Autodesk Fusion 360 part; units mm, degrees
(part 2 of 2)
sketch "Sketch9" plane through (0, 0, 3) normal (0, 0, 1) x (-1, 0, 0)
  line L0 (-28.8135, -26) -> (-30.5455, -23)
  line L1 (-30.5455, -23) -> (-28.8135, -20)
  line L2 (-28.8135, -20) -> (-25.3494, -20)
  line L3 (-25.3494, -20) -> (-23.6173, -23)
  line L4 (-23.6173, -23) -> (-25.3494, -26)
  line L5 (-25.3494, -26) -> (-28.8135, -26)
  line L6 (-28.8135, -33) -> (-30.5455, -30)
  line L7 (-30.5455, -30) -> (-28.8135, -27)
  line L8 (-28.8135, -27) -> (-25.3494, -27)
  line L9 (-25.3494, -27) -> (-23.6173, -30)
  line L10 (-23.6173, -30) -> (-25.3494, -33)
  line L11 (-25.3494, -33) -> (-28.8135, -33)
  line L12 (-34.8756, -29.5) -> (-36.6077, -26.5)
  line L13 (-36.6077, -26.5) -> (-34.8756, -23.5)
  line L14 (-34.8756, -23.5) -> (-31.4115, -23.5)
  line L15 (-31.4115, -23.5) -> (-29.6795, -26.5)
  line L16 (-29.6795, -26.5) -> (-31.4115, -29.5)
  line L17 (-31.4115, -29.5) -> (-34.8756, -29.5)
  line L18 (-40.9378, -26) -> (-42.6699, -23)
  line L19 (-42.6699, -23) -> (-40.9378, -20)
  line L20 (-40.9378, -20) -> (-37.4737, -20)
  line L21 (-37.4737, -20) -> (-35.7417, -23)
  line L22 (-35.7417, -23) -> (-37.4737, -26)
  line L23 (-37.4737, -26) -> (-40.9378, -26)
  line L24 (-34.8756, -22.5) -> (-36.6077, -19.5)
  line L25 (-36.6077, -19.5) -> (-34.8756, -16.5)
  line L26 (-34.8756, -16.5) -> (-31.4115, -16.5)
  line L27 (-31.4115, -16.5) -> (-29.6795, -19.5)
  line L28 (-29.6795, -19.5) -> (-31.4115, -22.5)
  line L29 (-31.4115, -22.5) -> (-34.8756, -22.5)
  line L30 (-47, -36.5) -> (-48.7321, -33.5)
  line L31 (-48.7321, -33.5) -> (-47, -30.5)
  line L32 (-47, -30.5) -> (-43.5359, -30.5)
  line L33 (-43.5359, -30.5) -> (-41.8038, -33.5)
  line L34 (-41.8038, -33.5) -> (-43.5359, -36.5)
  line L35 (-43.5359, -36.5) -> (-47, -36.5)
  line L36 (-40.9378, -12) -> (-42.6699, -9)
  line L37 (-42.6699, -9) -> (-40.9378, -6)
  line L38 (-40.9378, -6) -> (-37.4737, -6)
  line L39 (-37.4737, -6) -> (-35.7417, -9)
  line L40 (-35.7417, -9) -> (-37.4737, -12)
  line L41 (-37.4737, -12) -> (-40.9378, -12)
  line L42 (-47, -29.5) -> (-48.7321, -26.5)
  line L43 (-48.7321, -26.5) -> (-47, -23.5)
  line L44 (-47, -23.5) -> (-43.5359, -23.5)
  line L45 (-43.5359, -23.5) -> (-41.8038, -26.5)
  line L46 (-41.8038, -26.5) -> (-43.5359, -29.5)
  line L47 (-43.5359, -29.5) -> (-47, -29.5)
  line L48 (-10.6269, -8.5) -> (-12.359, -5.5)
  line L49 (-12.359, -5.5) -> (-10.6269, -2.5)
  line L50 (-10.6269, -2.5) -> (-7.1628, -2.5)
  line L51 (-7.1628, -2.5) -> (-5.4308, -5.5)
  line L52 (-5.4308, -5.5) -> (-7.1628, -8.5)
  line L53 (-7.1628, -8.5) -> (-10.6269, -8.5)
  line L54 (-10.6269, -15.5) -> (-12.359, -12.5)
  line L55 (-12.359, -12.5) -> (-10.6269, -9.5)
  line L56 (-10.6269, -9.5) -> (-7.1628, -9.5)
  line L57 (-7.1628, -9.5) -> (-5.4308, -12.5)
  line L58 (-5.4308, -12.5) -> (-7.1628, -15.5)
  line L59 (-7.1628, -15.5) -> (-10.6269, -15.5)
  line L60 (-10.6269, -29.5) -> (-12.359, -26.5)
  line L61 (-12.359, -26.5) -> (-10.6269, -23.5)
  line L62 (-10.6269, -23.5) -> (-7.1628, -23.5)
  line L63 (-7.1628, -23.5) -> (-5.4308, -26.5)
  line L64 (-5.4308, -26.5) -> (-7.1628, -29.5)
  line L65 (-7.1628, -29.5) -> (-10.6269, -29.5)
  line L66 (-40.9378, -33) -> (-42.6699, -30)
  line L67 (-42.6699, -30) -> (-40.9378, -27)
  line L68 (-40.9378, -27) -> (-37.4737, -27)
  line L69 (-37.4737, -27) -> (-35.7417, -30)
  line L70 (-35.7417, -30) -> (-37.4737, -33)
  line L71 (-37.4737, -33) -> (-40.9378, -33)
  line L72 (-22.7513, -15.5) -> (-24.4833, -12.5)
  line L73 (-24.4833, -12.5) -> (-22.7513, -9.5)
  line L74 (-22.7513, -9.5) -> (-19.2872, -9.5)
  line L75 (-19.2872, -9.5) -> (-17.5551, -12.5)
  line L76 (-17.5551, -12.5) -> (-19.2872, -15.5)
  line L77 (-19.2872, -15.5) -> (-22.7513, -15.5)
  line L78 (-34.8756, -15.5) -> (-36.6077, -12.5)
  line L79 (-36.6077, -12.5) -> (-34.8756, -9.5)
  line L80 (-34.8756, -9.5) -> (-31.4115, -9.5)
  line L81 (-31.4115, -9.5) -> (-29.6795, -12.5)
  line L82 (-29.6795, -12.5) -> (-31.4115, -15.5)
  line L83 (-31.4115, -15.5) -> (-34.8756, -15.5)
  line L84 (-28.8135, -12) -> (-30.5455, -9)
  line L85 (-30.5455, -9) -> (-28.8135, -6)
  line L86 (-28.8135, -6) -> (-25.3494, -6)
  line L87 (-25.3494, -6) -> (-23.6173, -9)
  line L88 (-23.6173, -9) -> (-25.3494, -12)
  line L89 (-25.3494, -12) -> (-28.8135, -12)
  line L90 (-47, -8.5) -> (-48.7321, -5.5)
  line L91 (-48.7321, -5.5) -> (-47, -2.5)
  line L92 (-47, -2.5) -> (-43.5359, -2.5)
  line L93 (-43.5359, -2.5) -> (-41.8038, -5.5)
  line L94 (-41.8038, -5.5) -> (-43.5359, -8.5)
  line L95 (-43.5359, -8.5) -> (-47, -8.5)
  line L96 (-34.8756, -36.5) -> (-36.6077, -33.5)
  line L97 (-36.6077, -33.5) -> (-34.8756, -30.5)
  line L98 (-34.8756, -30.5) -> (-31.4115, -30.5)
  line L99 (-31.4115, -30.5) -> (-29.6795, -33.5)
  line L100 (-29.6795, -33.5) -> (-31.4115, -36.5)
  line L101 (-31.4115, -36.5) -> (-34.8756, -36.5)
  line L102 (-16.6891, -19) -> (-18.4212, -16)
  line L103 (-18.4212, -16) -> (-16.6891, -13)
  line L104 (-16.6891, -13) -> (-13.225, -13)
  line L105 (-13.225, -13) -> (-11.493, -16)
  line L106 (-11.493, -16) -> (-13.225, -19)
  line L107 (-13.225, -19) -> (-16.6891, -19)
  line L108 (-22.7513, -22.5) -> (-24.4833, -19.5)
  line L109 (-24.4833, -19.5) -> (-22.7513, -16.5)
  line L110 (-22.7513, -16.5) -> (-19.2872, -16.5)
  line L111 (-19.2872, -16.5) -> (-17.5551, -19.5)
  line L112 (-17.5551, -19.5) -> (-19.2872, -22.5)
  line L113 (-19.2872, -22.5) -> (-22.7513, -22.5)
  line L114 (-16.6891, -12) -> (-18.4212, -9)
  line L115 (-18.4212, -9) -> (-16.6891, -6)
  line L116 (-16.6891, -6) -> (-13.225, -6)
  line L117 (-13.225, -6) -> (-11.493, -9)
  line L118 (-11.493, -9) -> (-13.225, -12)
  line L119 (-13.225, -12) -> (-16.6891, -12)
  line L120 (-10.6269, -36.5) -> (-12.359, -33.5)
  line L121 (-12.359, -33.5) -> (-10.6269, -30.5)
  line L122 (-10.6269, -30.5) -> (-7.1628, -30.5)
  line L123 (-7.1628, -30.5) -> (-5.4308, -33.5)
  line L124 (-5.4308, -33.5) -> (-7.1628, -36.5)
  line L125 (-7.1628, -36.5) -> (-10.6269, -36.5)
  line L126 (-10.6269, -22.5) -> (-12.359, -19.5)
  line L127 (-12.359, -19.5) -> (-10.6269, -16.5)
  line L128 (-10.6269, -16.5) -> (-7.1628, -16.5)
  line L129 (-7.1628, -16.5) -> (-5.4308, -19.5)
  line L130 (-5.4308, -19.5) -> (-7.1628, -22.5)
  line L131 (-7.1628, -22.5) -> (-10.6269, -22.5)
  line L132 (-40.9378, -19) -> (-42.6699, -16)
  line L133 (-42.6699, -16) -> (-40.9378, -13)
  line L134 (-40.9378, -13) -> (-37.4737, -13)
  line L135 (-37.4737, -13) -> (-35.7417, -16)
  line L136 (-35.7417, -16) -> (-37.4737, -19)
  line L137 (-37.4737, -19) -> (-40.9378, -19)
  line L138 (-47, -15.5) -> (-48.7321, -12.5)
  line L139 (-48.7321, -12.5) -> (-47, -9.5)
  line L140 (-47, -9.5) -> (-43.5359, -9.5)
  line L141 (-43.5359, -9.5) -> (-41.8038, -12.5)
  line L142 (-41.8038, -12.5) -> (-43.5359, -15.5)
  line L143 (-43.5359, -15.5) -> (-47, -15.5)
  line L144 (-16.6891, -33) -> (-18.4212, -30)
  line L145 (-18.4212, -30) -> (-16.6891, -27)
  line L146 (-16.6891, -27) -> (-13.225, -27)
  line L147 (-13.225, -27) -> (-11.493, -30)
  line L148 (-11.493, -30) -> (-13.225, -33)
  line L149 (-13.225, -33) -> (-16.6891, -33)
  line L150 (-16.6891, -26) -> (-18.4212, -23)
  line L151 (-18.4212, -23) -> (-16.6891, -20)
  line L152 (-16.6891, -20) -> (-13.225, -20)
  line L153 (-13.225, -20) -> (-11.493, -23)
  line L154 (-11.493, -23) -> (-13.225, -26)
  line L155 (-13.225, -26) -> (-16.6891, -26)
  line L156 (-47, -22.5) -> (-48.7321, -19.5)
  line L157 (-48.7321, -19.5) -> (-47, -16.5)
  line L158 (-47, -16.5) -> (-43.5359, -16.5)
  line L159 (-43.5359, -16.5) -> (-41.8038, -19.5)
  line L160 (-41.8038, -19.5) -> (-43.5359, -22.5)
  line L161 (-43.5359, -22.5) -> (-47, -22.5)
  line L162 (-22.7513, -36.5) -> (-24.4833, -33.5)
  line L163 (-24.4833, -33.5) -> (-22.7513, -30.5)
  line L164 (-22.7513, -30.5) -> (-19.2872, -30.5)
  line L165 (-19.2872, -30.5) -> (-17.5551, -33.5)
  line L166 (-17.5551, -33.5) -> (-19.2872, -36.5)
  line L167 (-19.2872, -36.5) -> (-22.7513, -36.5)
  line L168 (-34.8756, -8.5) -> (-36.6077, -5.5)
  line L169 (-36.6077, -5.5) -> (-34.8756, -2.5)
  line L170 (-34.8756, -2.5) -> (-31.4115, -2.5)
  line L171 (-31.4115, -2.5) -> (-29.6795, -5.5)
  line L172 (-29.6795, -5.5) -> (-31.4115, -8.5)
  line L173 (-31.4115, -8.5) -> (-34.8756, -8.5)
  line L174 (-22.7513, -29.5) -> (-24.4833, -26.5)
  line L175 (-24.4833, -26.5) -> (-22.7513, -23.5)
  line L176 (-22.7513, -23.5) -> (-19.2872, -23.5)
  line L177 (-19.2872, -23.5) -> (-17.5551, -26.5)
  line L178 (-17.5551, -26.5) -> (-19.2872, -29.5)
  line L179 (-19.2872, -29.5) -> (-22.7513, -29.5)
  line L180 (-22.7513, -8.5) -> (-24.4833, -5.5)
  line L181 (-24.4833, -5.5) -> (-22.7513, -2.5)
  line L182 (-22.7513, -2.5) -> (-19.2872, -2.5)
  line L183 (-19.2872, -2.5) -> (-17.5551, -5.5)
  line L184 (-17.5551, -5.5) -> (-19.2872, -8.5)
  line L185 (-19.2872, -8.5) -> (-22.7513, -8.5)
  line L186 (-28.8135, -19) -> (-30.5455, -16)
  line L187 (-30.5455, -16) -> (-28.8135, -13)
  line L188 (-28.8135, -13) -> (-25.3494, -13)
  line L189 (-25.3494, -13) -> (-23.6173, -16)
  line L190 (-23.6173, -16) -> (-25.3494, -19)
  line L191 (-25.3494, -19) -> (-28.8135, -19)
  line L192 (1, 1) -> (-57, 1)
  line L193 (-57, 1) -> (-57, -40)
  line L194 (-57, -40) -> (1, -40)
  line L195 (1, -40) -> (1, -37)
  line L196 (1, -37) -> (3, -37)
  line L197 (3, -37) -> (3, -2)
  line L198 (3, -2) -> (1, -2)
  line L199 (1, -2) -> (1, 1)
  line L200 (-55, -38) -> (-1, -38)
  line L201 (-1, -38) -> (-1, -1)
  line L202 (-1, -1) -> (-55, -1)
  line L203 (-55, -1) -> (-55, -38)
  constraint horizontal L200
  constraint vertical L201
  constraint horizontal L202
  constraint vertical L203
extrude "Extrude13" add sketch "Sketch9" along normal blind 2 contours L192 L193 L194 L195 L196 L197 L198 L199
extrude "Extrude14" cut 1 faces at (52.9107, 19.5, 3) along direction (0, 0, -1) blind 1
sketch "Sketch10" plane through (0, 0, 5) normal (0, 0, 1) x (-1, 0, 0)
  line L0 (-55, -38) -> (-55, -1)
  line L1 (-55, -1) -> (-1, -1)
  line L2 (-1, -1) -> (-1, -38)
  line L3 (-1, -38) -> (-55, -38)
  line L4 (1, -2) -> (1, 1)
  line L5 (1, 1) -> (-57, 1)
  line L6 (-57, 1) -> (-57, -40)
  line L7 (-57, -40) -> (1, -40)
  line L8 (1, -40) -> (1, -37)
  line L9 (1, -37) -> (3, -37)
  line L10 (3, -37) -> (3, -2)
  line L11 (3, -2) -> (1, -2)
  line L12 (0.5, -39.5) -> (-56.5, -39.5)
  line L13 (-56.5, -39.5) -> (-56.5, 0.5)
  line L14 (-56.5, 0.5) -> (0.5, 0.5)
  line L15 (3, -2) -> (0.5, -2)
  line L16 (0.5, -37) -> (3, -37)
  line L17 (3, -37) -> (3, -2)
  line L18 (0.5, 0.5) -> (0.5, -2)
  line L19 (0.5, -37) -> (0.5, -39.5)
  constraint horizontal L12
  constraint vertical L13
  constraint horizontal L14
  constraint vertical L18
  constraint horizontal L15
  constraint horizontal L16
  constraint vertical L17
  constraint coincident L16.start L18
  constraint coincident L10.end L11.start
  constraint collinear L18 L19
extrude "Extrude15" cut 1 faces at (37, 39.3333, 5) along direction (0, 0, -1) blind 3
extrude "Extrude16" add sketch "Sketch10" against normal blind 3 contours L9 L10 L11 L12 L13 L14 L15 L16 L17 L18 L19
